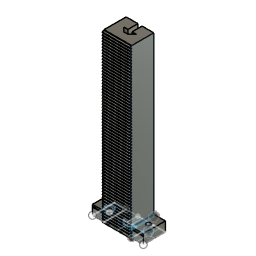
Rack_Gear_New_Version v6 (Autodesk Fusion 360 design; units mm, degrees)
description: Rack Gear; Module: 0.750000; Number of Teeth: 64; Pressure Angle: 20.000000; Root Fillet Radius: 0.032000; Clearance: 0.000000; Gear Thickness: 2.500000; Height: 2.000000;
Autodesk Fusion 360 part; units mm, degrees
(part 1 of 2)
sketch "Sketch1" plane through (0, 0, 0) normal (0, 1, 0) x (1, 0, 0) in component "Rack Gear (64 teeth)"
  line L0 (68.3534, 18.3125) -> (68.3059, 18.3125)
  arc A0 (75.3982, 18.3134) -> (75.0738, 18.5231) centre (75.3745, 18.6325) cw
  line L1 (63.641, 18.3125) -> (63.5935, 18.3125)
  arc A1 (63.5935, 18.3125) -> (63.2928, 18.5231) centre (63.5935, 18.6325) cw
  line L2 (62.7552, 20) -> (62.1231, 20)
  arc A2 (73.3665, 18.5231) -> (73.0658, 18.3125) centre (73.0658, 18.6325) cw
  arc A3 (71.0103, 18.5231) -> (70.7096, 18.3125) centre (70.7096, 18.6325) cw
  arc A4 (65.9497, 18.3125) -> (65.649, 18.5231) centre (65.9497, 18.6325) cw
  line L3 (74.5362, 20) -> (73.9041, 20)
  arc A5 (66.2979, 18.5231) -> (65.9972, 18.3125) centre (65.9972, 18.6325) cw
  line L4 (72.7176, 18.5231) -> (72.18, 20)
  arc A6 (70.6621, 18.3125) -> (70.3614, 18.5231) centre (70.6621, 18.6325) cw
  line L5 (63.2928, 18.5231) -> (62.7552, 20)
  line L6 (73.0658, 18.3125) -> (73.0183, 18.3125)
  line L7 (69.8238, 20) -> (69.1917, 20)
  line L8 (65.1114, 20) -> (64.4793, 20)
  line L9 (65.649, 18.5231) -> (65.1114, 20)
  line L10 (64.4793, 20) -> (63.9417, 18.5231)
  line L11 (70.7096, 18.3125) -> (70.6621, 18.3125)
  line L12 (68.0052, 18.5231) -> (67.4676, 20)
  arc A7 (73.0183, 18.3125) -> (72.7176, 18.5231) centre (73.0183, 18.6325) cw
  line L13 (67.4676, 20) -> (66.8355, 20)
  arc A8 (68.6541, 18.5231) -> (68.3534, 18.3125) centre (68.3534, 18.6325) cw
  line L14 (72.18, 20) -> (71.5479, 20)
  line L15 (75.0738, 18.5231) -> (74.5362, 20)
  arc A9 (68.3059, 18.3125) -> (68.0052, 18.5231) centre (68.3059, 18.6325) cw
  line L16 (71.5479, 20) -> (71.0103, 18.5231)
  line L17 (66.8355, 20) -> (66.2979, 18.5231)
  line L18 (65.9972, 18.3125) -> (65.9497, 18.3125)
  arc A10 (58.8811, 18.3125) -> (58.5804, 18.5231) centre (58.8811, 18.6325) cw
  line L19 (42.087, 18.5231) -> (41.5495, 20)
  arc A11 (63.9417, 18.5231) -> (63.641, 18.3125) centre (63.641, 18.6325) cw
  line L20 (73.9041, 20) -> (73.3665, 18.5231)
  line L21 (70.3614, 18.5231) -> (69.8238, 20)
  line L22 (69.1917, 20) -> (68.6541, 18.5231)
  line L23 (39.7308, 18.5231) -> (39.1933, 20)
  line L24 (40.9173, 20) -> (40.3798, 18.5231)
  arc A12 (49.4563, 18.3125) -> (49.1556, 18.5231) centre (49.4563, 18.6325) cw
  line L25 (58.5804, 18.5231) -> (58.0428, 20)
  arc A13 (40.0315, 18.3125) -> (39.7308, 18.5231) centre (40.0315, 18.6325) cw
  line L26 (46.2619, 20) -> (45.6297, 20)
  arc A14 (54.5169, 18.5231) -> (54.2162, 18.3125) centre (54.2162, 18.6325) cw
  line L27 (40.0791, 18.3125) -> (40.0315, 18.3125)
  line L28 (50.9743, 20) -> (50.3421, 20)
  line L29 (39.1933, 20) -> (38.5611, 20)
  arc A15 (38.0236, 18.5231) -> (37.7229, 18.3125) centre (37.7229, 18.6325) cw
  arc A16 (54.1687, 18.3125) -> (53.868, 18.5231) centre (54.1687, 18.6325) cw
  arc A17 (44.7439, 18.3125) -> (44.4432, 18.5231) centre (44.7439, 18.6325) cw
  arc A18 (37.6754, 18.3125) -> (37.3747, 18.5231) centre (37.6754, 18.6325) cw
  line L30 (37.7229, 18.3125) -> (37.6754, 18.3125)
  line L31 (55.6866, 20) -> (55.0545, 20)
  arc A19 (47.4484, 18.5231) -> (47.1477, 18.3125) centre (47.1476, 18.6325) cw
  line L32 (56.5724, 18.3125) -> (56.5249, 18.3125)
  line L33 (42.4353, 18.3125) -> (42.3877, 18.3125)
  line L34 (52.6983, 20) -> (52.1607, 18.5231)
  line L35 (53.868, 18.5231) -> (53.3304, 20)
  line L36 (57.4107, 20) -> (56.8731, 18.5231)
  line L37 (48.6181, 20) -> (47.9859, 20)
  line L38 (60.399, 20) -> (59.7669, 20)
  line L39 (43.2735, 20) -> (42.736, 18.5231)
  line L40 (45.6297, 20) -> (45.0922, 18.5231)
  arc A20 (61.2373, 18.3125) -> (60.9366, 18.5231) centre (61.2373, 18.6325) cw
  line L41 (44.4432, 18.5231) -> (43.9057, 20)
  line L42 (49.5038, 18.3125) -> (49.4563, 18.3125)
  arc A21 (42.736, 18.5231) -> (42.4353, 18.3125) centre (42.4353, 18.6325) cw
  line L43 (41.5495, 20) -> (40.9173, 20)
  line L44 (49.1556, 18.5231) -> (48.6181, 20)
  arc A22 (56.5249, 18.3125) -> (56.2242, 18.5231) centre (56.5249, 18.6325) cw
  arc A23 (51.8125, 18.3125) -> (51.5118, 18.5231) centre (51.8125, 18.6325) cw
  arc A24 (59.2293, 18.5231) -> (58.9286, 18.3125) centre (58.9286, 18.6325) cw
  line L45 (62.1231, 20) -> (61.5855, 18.5231)
  arc A25 (61.5855, 18.5231) -> (61.2848, 18.3125) centre (61.2848, 18.6325) cw
  line L46 (54.2162, 18.3125) -> (54.1687, 18.3125)
  line L47 (38.5611, 20) -> (38.0236, 18.5231)
  line L48 (51.5118, 18.5231) -> (50.9743, 20)
  line L49 (60.9366, 18.5231) -> (60.399, 20)
  line L50 (61.2848, 18.3125) -> (61.2373, 18.3125)
  line L51 (47.9859, 20) -> (47.4484, 18.5231)
  line L52 (56.2242, 18.5231) -> (55.6866, 20)
  line L53 (59.7669, 20) -> (59.2293, 18.5231)
  arc A26 (45.0922, 18.5231) -> (44.7915, 18.3125) centre (44.7915, 18.6325) cw
  arc A27 (47.1001, 18.3125) -> (46.7994, 18.5231) centre (47.1001, 18.6325) cw
  line L54 (47.1477, 18.3125) -> (47.1001, 18.3125)
  arc A28 (42.3877, 18.3125) -> (42.087, 18.5231) centre (42.3877, 18.6325) cw
  line L55 (58.9286, 18.3125) -> (58.8811, 18.3125)
  line L56 (32.1247, 20) -> (31.4926, 20)
  line L57 (51.86, 18.3125) -> (51.8125, 18.3125)
  arc A29 (40.3798, 18.5231) -> (40.0791, 18.3125) centre (40.0791, 18.6325) cw
  line L58 (44.7915, 18.3125) -> (44.7439, 18.3125)
  arc A30 (49.8045, 18.5231) -> (49.5038, 18.3125) centre (49.5038, 18.6325) cw
  line L59 (46.7994, 18.5231) -> (46.2619, 20)
  line L60 (55.0545, 20) -> (54.5169, 18.5231)
  arc A31 (52.1607, 18.5231) -> (51.86, 18.3125) centre (51.86, 18.6325) cw
  arc A32 (56.8731, 18.5231) -> (56.5724, 18.3125) centre (56.5724, 18.6325) cw
  line L61 (53.3304, 20) -> (52.6983, 20)
  line L62 (58.0428, 20) -> (57.4107, 20)
  line L63 (43.9057, 20) -> (43.2735, 20)
  line L64 (29.1364, 20) -> (28.5988, 18.5231)
  line L65 (50.3421, 20) -> (49.8045, 18.5231)
  line L66 (25.0561, 20) -> (24.424, 20)
  line L67 (24.424, 20) -> (23.8864, 18.5231)
  arc A33 (21.5302, 18.5231) -> (21.2295, 18.3125) centre (21.2295, 18.6325) cw
  arc A34 (30.955, 18.5231) -> (30.6543, 18.3125) centre (30.6543, 18.6325) cw
  line L68 (23.2375, 18.5231) -> (22.6999, 20)
  line L69 (20.8813, 18.5231) -> (20.3437, 20)
  arc A35 (35.3192, 18.3125) -> (35.0185, 18.5231) centre (35.3192, 18.6325) cw
  line L70 (37.3747, 18.5231) -> (36.8371, 20)
  line L71 (13.2751, 20) -> (12.643, 20)
  arc A36 (33.3112, 18.5231) -> (33.0105, 18.3125) centre (33.0105, 18.6325) cw
  arc A37 (14.1134, 18.3125) -> (13.8127, 18.5231) centre (14.1134, 18.6325) cw
  line L72 (28.2981, 18.3125) -> (28.2506, 18.3125)
  arc A38 (35.6674, 18.5231) -> (35.3667, 18.3125) centre (35.3667, 18.6325) cw
  line L73 (19.7116, 20) -> (19.174, 18.5231)
  arc A39 (21.182, 18.3125) -> (20.8813, 18.5231) centre (21.182, 18.6325) cw
  arc A40 (18.8258, 18.3125) -> (18.5251, 18.5231) centre (18.8258, 18.6325) cw
  line L74 (33.0105, 18.3125) -> (32.963, 18.3125)
  line L75 (26.7802, 20) -> (26.2426, 18.5231)
  arc A41 (16.8178, 18.5231) -> (16.5171, 18.3125) centre (16.5171, 18.6325) cw
  line L76 (15.6313, 20) -> (14.9992, 20)
  arc A42 (16.4696, 18.3125) -> (16.1689, 18.5231) centre (16.4696, 18.6325) cw
  arc A43 (30.6068, 18.3125) -> (30.3061, 18.5231) centre (30.6068, 18.6325) cw
  line L77 (25.9419, 18.3125) -> (25.8944, 18.3125)
  arc A44 (28.2506, 18.3125) -> (27.9499, 18.5231) centre (28.2506, 18.6325) cw
  line L78 (17.3554, 20) -> (16.8178, 18.5231)
  line L79 (36.2049, 20) -> (35.6674, 18.5231)
  line L80 (12.643, 20) -> (12.1054, 18.5231)
  line L81 (34.4809, 20) -> (33.8487, 20)
  arc A45 (25.8944, 18.3125) -> (25.5937, 18.5231) centre (25.8944, 18.6325) cw
  line L82 (35.3667, 18.3125) -> (35.3192, 18.3125)
  line L83 (29.7685, 20) -> (29.1364, 20)
  arc A46 (26.2426, 18.5231) -> (25.9419, 18.3125) centre (25.9419, 18.6325) cw
  arc A47 (12.1054, 18.5231) -> (11.8047, 18.3125) centre (11.8047, 18.6325) cw
  line L84 (23.5857, 18.3125) -> (23.5382, 18.3125)
  line L85 (33.8487, 20) -> (33.3112, 18.5231)
  line L86 (18.8733, 18.3125) -> (18.8258, 18.3125)
  line L87 (18.5251, 18.5231) -> (17.9875, 20)
  line L88 (13.8127, 18.5231) -> (13.2751, 20)
  arc A48 (23.8864, 18.5231) -> (23.5857, 18.3125) centre (23.5857, 18.6325) cw
  line L89 (16.1689, 18.5231) -> (15.6313, 20)
  line L90 (36.8371, 20) -> (36.2049, 20)
  line L91 (14.9992, 20) -> (14.4616, 18.5231)
  arc A49 (23.5382, 18.3125) -> (23.2375, 18.5231) centre (23.5382, 18.6325) cw
  line L92 (25.5937, 18.5231) -> (25.0561, 20)
  line L93 (21.2295, 18.3125) -> (21.182, 18.3125)
  line L94 (14.1609, 18.3125) -> (14.1134, 18.3125)
  line L95 (22.6999, 20) -> (22.0678, 20)
  arc A50 (32.963, 18.3125) -> (32.6623, 18.5231) centre (32.963, 18.6325) cw
  line L96 (32.6623, 18.5231) -> (32.1247, 20)
  line L97 (31.4926, 20) -> (30.955, 18.5231)
  line L98 (10.9189, 20) -> (10.2868, 20)
  arc A51 (2.6807, 18.5231) -> (2.38, 18.3125) centre (2.38, 18.6325) cw
  line L99 (30.3061, 18.5231) -> (29.7685, 20)
  line L100 (27.4123, 20) -> (26.7802, 20)
  line L101 (30.6543, 18.3125) -> (30.6068, 18.3125)
  line L102 (35.0185, 18.5231) -> (34.4809, 20)
  line L103 (22.0678, 20) -> (21.5302, 18.5231)
  arc A52 (28.5988, 18.5231) -> (28.2981, 18.3125) centre (28.2981, 18.6325) cw
  arc A53 (19.174, 18.5231) -> (18.8733, 18.3125) centre (18.8733, 18.6325) cw
  line L104 (20.3437, 20) -> (19.7116, 20)
  arc A54 (14.4616, 18.5231) -> (14.1609, 18.3125) centre (14.1609, 18.6325) cw
  line L105 (-7.9306, 20) -> (-8.5628, 20)
  arc A55 (11.7572, 18.3125) -> (11.4565, 18.5231) centre (11.7572, 18.6325) cw
  line L106 (16.5171, 18.3125) -> (16.4696, 18.3125)
  arc A56 (-9.1003, 18.5231) -> (-9.401, 18.3125) centre (-9.401, 18.6325) cw
  line L107 (-7.393, 18.5231) -> (-7.9306, 20)
  line L108 (2.38, 18.3125) -> (2.3324, 18.3125)
  line L109 (27.9499, 18.5231) -> (27.4123, 20)
  line L110 (17.9875, 20) -> (17.3554, 20)
  line L111 (10.2868, 20) -> (9.7492, 18.5231)
  line L112 (-0.862, 20) -> (-1.4942, 20)
  line L113 (-9.401, 18.3125) -> (-9.4485, 18.3125)
  arc A57 (-9.4485, 18.3125) -> (-9.7492, 18.5231) centre (-9.4485, 18.6325) cw
  arc A58 (-4.7361, 18.3125) -> (-5.0369, 18.5231) centre (-4.7361, 18.6325) cw
  line L114 (-10.2868, 20) -> (-10.9189, 20)
  arc A59 (-2.0317, 18.5231) -> (-2.3324, 18.3125) centre (-2.3324, 18.6325) cw
  line L115 (11.8047, 18.3125) -> (11.7572, 18.3125)
  line L116 (6.7441, 18.5231) -> (6.2066, 20)
  line L117 (-11.7572, 18.3125) -> (-11.8047, 18.3125)
  line L118 (7.0923, 18.3125) -> (7.0448, 18.3125)
  line L119 (-8.5628, 20) -> (-9.1003, 18.5231)
  line L120 (-7.0448, 18.3125) -> (-7.0923, 18.3125)
  line L121 (2.0317, 18.5231) -> (1.4942, 20)
  line L122 (4.7361, 18.3125) -> (4.6886, 18.3125)
  arc A60 (-0.0238, 18.3125) -> (-0.3245, 18.5231) centre (-0.0238, 18.6325) cw
  line L123 (-2.3324, 18.3125) -> (-2.38, 18.3125)
  arc A61 (9.7492, 18.5231) -> (9.4485, 18.3125) centre (9.4485, 18.6325) cw
  line L124 (-12.1054, 18.5231) -> (-12.643, 20)
  line L125 (-5.5744, 20) -> (-6.2066, 20)
  line L126 (-9.7492, 18.5231) -> (-10.2868, 20)
  line L127 (11.4565, 18.5231) -> (10.9189, 20)
  line L128 (-0.3245, 18.5231) -> (-0.862, 20)
  line L129 (-12.643, 20) -> (-13.2751, 20)
  line L130 (1.4942, 20) -> (0.862, 20)
  line L131 (-3.2182, 20) -> (-3.8504, 20)
  arc A62 (-4.3879, 18.5231) -> (-4.6886, 18.3125) centre (-4.6886, 18.6325) cw
  line L132 (-10.9189, 20) -> (-11.4565, 18.5231)
  arc A63 (-11.4565, 18.5231) -> (-11.7572, 18.3125) centre (-11.7572, 18.6325) cw
  line L133 (6.2066, 20) -> (5.5744, 20)
  arc A64 (4.6886, 18.3125) -> (4.3879, 18.5231) centre (4.6886, 18.6325) cw
  line L134 (0.0238, 18.3125) -> (-0.0238, 18.3125)
  line L135 (0.862, 20) -> (0.3245, 18.5231)
  line L136 (9.4485, 18.3125) -> (9.401, 18.3125)
  arc A65 (-11.8047, 18.3125) -> (-12.1054, 18.5231) centre (-11.8047, 18.6325) cw
  line L137 (5.5744, 20) -> (5.0369, 18.5231)
  line L138 (4.3879, 18.5231) -> (3.8504, 20)
  line L139 (3.8504, 20) -> (3.2182, 20)
  arc A66 (9.401, 18.3125) -> (9.1003, 18.5231) centre (9.401, 18.6325) cw
  line L140 (-1.4942, 20) -> (-2.0317, 18.5231)
  line L141 (7.9306, 20) -> (7.393, 18.5231)
  line L142 (-4.6886, 18.3125) -> (-4.7361, 18.3125)
  arc A67 (-6.7441, 18.5231) -> (-7.0448, 18.3125) centre (-7.0448, 18.6325) cw
  arc A68 (7.0448, 18.3125) -> (6.7441, 18.5231) centre (7.0448, 18.6325) cw
  arc A69 (7.393, 18.5231) -> (7.0923, 18.3125) centre (7.0923, 18.6325) cw
  arc A70 (0.3245, 18.5231) -> (0.0238, 18.3125) centre (0.0238, 18.6325) cw
  line L143 (-6.2066, 20) -> (-6.7441, 18.5231)
  line L144 (-3.8504, 20) -> (-4.3879, 18.5231)
  arc A71 (-7.0923, 18.3125) -> (-7.393, 18.5231) centre (-7.0923, 18.6325) cw
  arc A72 (5.0369, 18.5231) -> (4.7361, 18.3125) centre (4.7361, 18.6325) cw
  line L145 (9.1003, 18.5231) -> (8.5628, 20)
  arc A73 (-2.38, 18.3125) -> (-2.6807, 18.5231) centre (-2.38, 18.6325) cw
  line L146 (-2.6807, 18.5231) -> (-3.2182, 20)
  line L147 (-5.0369, 18.5231) -> (-5.5744, 20)
  line L148 (3.2182, 20) -> (2.6807, 18.5231)
  arc A74 (2.3324, 18.3125) -> (2.0317, 18.5231) centre (2.3324, 18.6325) cw
  line L149 (8.5628, 20) -> (7.9306, 20)
  arc A75 (-23.2375, 18.5231) -> (-23.5382, 18.3125) centre (-23.5382, 18.6325) cw
  line L150 (-19.7116, 20) -> (-20.3437, 20)
  line L151 (-25.8944, 18.3125) -> (-25.9419, 18.3125)
  arc A76 (-16.1689, 18.5231) -> (-16.4696, 18.3125) centre (-16.4696, 18.6325) cw
  line L152 (-33.3112, 18.5231) -> (-33.8487, 20)
  arc A77 (-16.5171, 18.3125) -> (-16.8178, 18.5231) centre (-16.5171, 18.6325) cw
  arc A78 (-37.7229, 18.3125) -> (-38.0236, 18.5231) centre (-37.7229, 18.6325) cw
  line L153 (-36.2049, 20) -> (-36.8371, 20)
  line L154 (-17.9875, 20) -> (-18.5251, 18.5231)
  line L155 (-26.7802, 20) -> (-27.4123, 20)
  line L156 (-20.3437, 20) -> (-20.8813, 18.5231)
  arc A79 (-27.9499, 18.5231) -> (-28.2506, 18.3125) centre (-28.2506, 18.6325) cw
  line L157 (-26.2426, 18.5231) -> (-26.7802, 20)
  arc A80 (-28.2981, 18.3125) -> (-28.5988, 18.5231) centre (-28.2981, 18.6325) cw
  line L158 (-30.6068, 18.3125) -> (-30.6543, 18.3125)
  line L159 (-21.182, 18.3125) -> (-21.2295, 18.3125)
  line L160 (-25.0561, 20) -> (-25.5937, 18.5231)
  line L161 (-34.4809, 20) -> (-35.0185, 18.5231)
  line L162 (-35.3192, 18.3125) -> (-35.3667, 18.3125)
  line L163 (-14.1134, 18.3125) -> (-14.1609, 18.3125)
  arc A81 (-20.8813, 18.5231) -> (-21.182, 18.3125) centre (-21.182, 18.6325) cw
  line L164 (-14.9992, 20) -> (-15.6313, 20)
  arc A82 (-18.8733, 18.3125) -> (-19.174, 18.5231) centre (-18.8733, 18.6325) cw
  line L165 (-23.8864, 18.5231) -> (-24.424, 20)
  arc A83 (-23.5857, 18.3125) -> (-23.8864, 18.5231) centre (-23.5857, 18.6325) cw
  arc A84 (-56.5724, 18.3125) -> (-56.8731, 18.5231) centre (-56.5724, 18.6325) cw
  arc A85 (-21.2295, 18.3125) -> (-21.5302, 18.5231) centre (-21.2295, 18.6325) cw
  line L166 (-31.4926, 20) -> (-32.1247, 20)
  line L167 (-22.6999, 20) -> (-23.2375, 18.5231)
  line L168 (-24.424, 20) -> (-25.0561, 20)
  line L169 (-15.6313, 20) -> (-16.1689, 18.5231)
  arc A86 (-25.9419, 18.3125) -> (-26.2426, 18.5231) centre (-25.9419, 18.6325) cw
  line L170 (-17.3554, 20) -> (-17.9875, 20)
  line L171 (-16.4696, 18.3125) -> (-16.5171, 18.3125)
  line L172 (-36.8371, 20) -> (-37.3747, 18.5231)
  arc A87 (-14.1609, 18.3125) -> (-14.4616, 18.5231) centre (-14.1609, 18.6325) cw
  line L173 (-13.2751, 20) -> (-13.8127, 18.5231)
  arc A88 (-30.3061, 18.5231) -> (-30.6068, 18.3125) centre (-30.6068, 18.6325) cw
  line L174 (-21.5302, 18.5231) -> (-22.0678, 20)
  line L175 (-22.0678, 20) -> (-22.6999, 20)
  line L176 (-32.963, 18.3125) -> (-33.0105, 18.3125)
  arc A89 (-13.8127, 18.5231) -> (-14.1134, 18.3125) centre (-14.1134, 18.6325) cw
  line L177 (-37.6754, 18.3125) -> (-37.7229, 18.3125)
  line L178 (-48.6181, 20) -> (-49.1556, 18.5231)
  line L179 (-59.2293, 18.5231) -> (-59.7669, 20)
  line L180 (-32.1247, 20) -> (-32.6623, 18.5231)
  line L181 (-18.8258, 18.3125) -> (-18.8733, 18.3125)
  line L182 (-45.0922, 18.5231) -> (-45.6297, 20)
  line L183 (-33.8487, 20) -> (-34.4809, 20)
  line L184 (-55.6866, 20) -> (-56.2242, 18.5231)
  arc A90 (-32.6623, 18.5231) -> (-32.963, 18.3125) centre (-32.963, 18.6325) cw
  line L185 (-23.5382, 18.3125) -> (-23.5857, 18.3125)
  line L186 (-16.8178, 18.5231) -> (-17.3554, 20)
  line L187 (-29.1364, 20) -> (-29.7685, 20)
  arc A91 (-33.0105, 18.3125) -> (-33.3112, 18.5231) centre (-33.0105, 18.6325) cw
  arc A92 (-30.6543, 18.3125) -> (-30.955, 18.5231) centre (-30.6543, 18.6325) cw
  line L188 (-14.4616, 18.5231) -> (-14.9992, 20)
  line L189 (-29.7685, 20) -> (-30.3061, 18.5231)
  line L190 (-28.5988, 18.5231) -> (-29.1364, 20)
  line L191 (-35.6674, 18.5231) -> (-36.2049, 20)
  arc A93 (-37.3747, 18.5231) -> (-37.6754, 18.3125) centre (-37.6754, 18.6325) cw
  line L192 (-28.2506, 18.3125) -> (-28.2981, 18.3125)
  arc A94 (-35.3667, 18.3125) -> (-35.6674, 18.5231) centre (-35.3667, 18.6325) cw
  line L193 (-30.955, 18.5231) -> (-31.4926, 20)
  arc A95 (-25.5937, 18.5231) -> (-25.8944, 18.3125) centre (-25.8944, 18.6325) cw
  line L194 (-19.174, 18.5231) -> (-19.7116, 20)
  arc A96 (-35.0185, 18.5231) -> (-35.3192, 18.3125) centre (-35.3192, 18.6325) cw
  line L195 (-27.4123, 20) -> (-27.9499, 18.5231)
  arc A97 (-49.5038, 18.3125) -> (-49.8045, 18.5231) centre (-49.5038, 18.6325) cw
  arc A98 (-58.9286, 18.3125) -> (-59.2293, 18.5231) centre (-58.9286, 18.6325) cw
  arc A99 (-18.5251, 18.5231) -> (-18.8258, 18.3125) centre (-18.8258, 18.6325) cw
  line L196 (-59.7669, 20) -> (-60.399, 20)
  line L197 (-54.5169, 18.5231) -> (-55.0545, 20)
  arc A100 (-60.9366, 18.5231) -> (-61.2373, 18.3125) centre (-61.2373, 18.6325) cw
  arc A101 (-58.5804, 18.5231) -> (-58.8811, 18.3125) centre (-58.8811, 18.6325) cw
  arc A102 (-42.087, 18.5231) -> (-42.3877, 18.3125) centre (-42.3877, 18.6325) cw
  arc A103 (-47.1477, 18.3125) -> (-47.4484, 18.5231) centre (-47.1476, 18.6325) cw
  line L198 (-45.6297, 20) -> (-46.2619, 20)
  arc A104 (-49.1556, 18.5231) -> (-49.4563, 18.3125) centre (-49.4563, 18.6325) cw
  arc A105 (-51.86, 18.3125) -> (-52.1607, 18.5231) centre (-51.86, 18.6325) cw
  line L199 (-54.1687, 18.3125) -> (-54.2162, 18.3125)
  line L200 (-50.9743, 20) -> (-51.5118, 18.5231)
  line L201 (-56.8731, 18.5231) -> (-57.4107, 20)
  line L202 (-58.8811, 18.3125) -> (-58.9286, 18.3125)
  arc A106 (-61.2848, 18.3125) -> (-61.5855, 18.5231) centre (-61.2848, 18.6325) cw
  line L203 (-61.2373, 18.3125) -> (-61.2848, 18.3125)
  arc A107 (-44.7915, 18.3125) -> (-45.0922, 18.5231) centre (-44.7915, 18.6325) cw
  line L204 (-52.6983, 20) -> (-53.3304, 20)
  arc A108 (-63.2928, 18.5231) -> (-63.5935, 18.3125) centre (-63.5935, 18.6325) cw
  line L205 (-43.9057, 20) -> (-44.4432, 18.5231)
  line L206 (-47.9859, 20) -> (-48.6181, 20)
  line L207 (-61.5855, 18.5231) -> (-62.1231, 20)
  line L208 (-58.0428, 20) -> (-58.5804, 18.5231)
  arc A109 (-42.4353, 18.3125) -> (-42.736, 18.5231) centre (-42.4353, 18.6325) cw
  arc A110 (-53.868, 18.5231) -> (-54.1687, 18.3125) centre (-54.1687, 18.6325) cw
  line L209 (-55.0545, 20) -> (-55.6866, 20)
  line L210 (-40.9173, 20) -> (-41.5495, 20)
  line L211 (-42.736, 18.5231) -> (-43.2735, 20)
  line L212 (-42.3877, 18.3125) -> (-42.4353, 18.3125)
  line L213 (-47.4484, 18.5231) -> (-47.9859, 20)
  line L214 (-40.0315, 18.3125) -> (-40.0791, 18.3125)
  line L215 (-41.5495, 20) -> (-42.087, 18.5231)
  line L216 (-38.0236, 18.5231) -> (-38.5611, 20)
  arc A111 (-54.2162, 18.3125) -> (-54.5169, 18.5231) centre (-54.2162, 18.6325) cw
  line L217 (-49.4563, 18.3125) -> (-49.5038, 18.3125)
  arc A112 (-56.2242, 18.5231) -> (-56.5249, 18.3125) centre (-56.5249, 18.6325) cw
  line L218 (-40.3798, 18.5231) -> (-40.9173, 20)
  line L219 (-44.7439, 18.3125) -> (-44.7915, 18.3125)
  line L220 (-52.1607, 18.5231) -> (-52.6983, 20)
  arc A113 (-39.7308, 18.5231) -> (-40.0315, 18.3125) centre (-40.0315, 18.6325) cw
  line L221 (-43.2735, 20) -> (-43.9057, 20)
  line L222 (-60.399, 20) -> (-60.9366, 18.5231)
  arc A114 (-51.5118, 18.5231) -> (-51.8125, 18.3125) centre (-51.8125, 18.6325) cw
  line L223 (-50.3421, 20) -> (-50.9743, 20)
  line L224 (-62.1231, 20) -> (-62.7552, 20)
  line L225 (-62.7552, 20) -> (-63.2928, 18.5231)
  arc A115 (-44.4432, 18.5231) -> (-44.7439, 18.3125) centre (-44.7439, 18.6325) cw
  line L226 (-49.8045, 18.5231) -> (-50.3421, 20)
  line L227 (-56.5249, 18.3125) -> (-56.5724, 18.3125)
  line L228 (-51.8125, 18.3125) -> (-51.86, 18.3125)
  line L229 (-38.5611, 20) -> (-39.1933, 20)
  arc A116 (-65.9972, 18.3125) -> (-66.2979, 18.5231) centre (-65.9972, 18.6325) cw
  line L230 (-72.18, 20) -> (-72.7176, 18.5231)
  arc A117 (-65.649, 18.5231) -> (-65.9497, 18.3125) centre (-65.9497, 18.6325) cw
  line L231 (-73.9041, 20) -> (-74.5362, 20)
  line L232 (-46.2619, 20) -> (-46.7994, 18.5231)
  line L233 (-66.2979, 18.5231) -> (-66.8355, 20)
  line L234 (-73.3665, 18.5231) -> (-73.9041, 20)
  line L235 (-73.0183, 18.3125) -> (-73.0658, 18.3125)
  arc A118 (-63.641, 18.3125) -> (-63.9417, 18.5231) centre (-63.641, 18.6325) cw
  line L236 (-70.6621, 18.3125) -> (-70.7096, 18.3125)
  line L237 (-74.5362, 20) -> (-75.0738, 18.5231)
  line L238 (-53.3304, 20) -> (-53.868, 18.5231)
  arc A119 (-75.0738, 18.5231) -> (-75.3982, 18.3134) centre (-75.3745, 18.6325) cw
  line L239 (-65.1114, 20) -> (-65.649, 18.5231)
  line L240 (-71.0103, 18.5231) -> (-71.5479, 20)
  arc A120 (-46.7994, 18.5231) -> (-47.1001, 18.3125) centre (-47.1001, 18.6325) cw
  arc A121 (-70.7096, 18.3125) -> (-71.0103, 18.5231) centre (-70.7096, 18.6325) cw
  line L241 (-47.1001, 18.3125) -> (-47.1477, 18.3125)
  line L242 (-63.5935, 18.3125) -> (-63.641, 18.3125)
  line L243 (-67.4676, 20) -> (-68.0052, 18.5231)
  line L244 (-68.6541, 18.5231) -> (-69.1917, 20)
  line L245 (-69.8238, 20) -> (-70.3614, 18.5231)
  line L246 (-63.9417, 18.5231) -> (-64.4793, 20)
  line L247 (-64.4793, 20) -> (-65.1114, 20)
  line L248 (-75.3982, 0) -> (75.3982, 0)
  line L249 (-65.9497, 18.3125) -> (-65.9972, 18.3125)
  arc A122 (-68.3534, 18.3125) -> (-68.6541, 18.5231) centre (-68.3534, 18.6325) cw
  arc A123 (-68.0052, 18.5231) -> (-68.3059, 18.3125) centre (-68.3059, 18.6325) cw
  line L250 (-69.1917, 20) -> (-69.8238, 20)
  line L251 (-57.4107, 20) -> (-58.0428, 20)
  line L252 (-71.5479, 20) -> (-72.18, 20)
  line L253 (-39.1933, 20) -> (-39.7308, 18.5231)
  arc A124 (-73.0658, 18.3125) -> (-73.3665, 18.5231) centre (-73.0658, 18.6325) cw
  arc A125 (-40.0791, 18.3125) -> (-40.3798, 18.5231) centre (-40.0791, 18.6325) cw
  line L254 (-66.8355, 20) -> (-67.4676, 20)
  arc A126 (-72.7176, 18.5231) -> (-73.0183, 18.3125) centre (-73.0183, 18.6325) cw
  line L255 (-75.3982, 18.3134) -> (-75.3982, 0)
  line L256 (-68.3059, 18.3125) -> (-68.3534, 18.3125)
  arc A127 (-70.3614, 18.5231) -> (-70.6621, 18.3125) centre (-70.6621, 18.6325) cw
  line L257 (75.3982, 0) -> (75.3982, 18.3134)
extrude "Extrude1" add sketch "Sketch1" along normal blind 25 makes body 1 in component "Rack Gear (64 teeth)"
sketch "Sketch2" plane through (0, 0, 0) normal (0, 1, 0) x (1, 0, 0) in component "Rack Gear (64 teeth)"
  line L0 (-75.4082, 19.25) -> (75.4082, 19.25) construction
extrude "Extrude2" add 1 faces at (-25.1327, 16.6667, 0) along direction (0, 0, 1) blind 1.687 on bodies 1 bodies 1 in component "Rack Gear (64 teeth)"
sketch "Sketch1 (2)" plane through (0, 0, -86.9185) normal (0, 0, -1) x (1, 0, 0)
  line L0 (12.5, -25.7073) -> (12.5, -5.707)
  line L1 (12.5, -5.707) -> (-12.5, -5.707)
  line L2 (-12.5, -5.707) -> (-12.5, -25.7073)
  line L3 (-12.5, -25.7073) -> (12.5, -25.7073)
  line L4 (12.5, -5.707) -> (-12.5, -5.707) construction
  line L5 (-12.5, -5.707) -> (-12.5, -25.7073) construction
  line L6 (-12.5, -25.7073) -> (12.5, -25.7073) construction
  line L7 (12.5, -25.7073) -> (12.5, -5.707) construction
  line L8 (0, -25.7073) -> (0, -5.707)
  line L9 (-12.5, -15.7072) -> (12.5, -15.7072)
  line L10 (23, -25.7073) -> (23, -5.707) construction
  line L11 (12.5, -5.707) -> (23, -5.707)
  line L12 (23, -5.707) -> (23, -25.7073)
  line L13 (23, -25.7073) -> (12.5, -25.7073)
  line L14 (12.5, -25.7073) -> (12.5, -5.707)
  line L15 (-12.5, -5.707) -> (-23, -5.707)
  line L16 (-23, -25.7073) -> (-23, -5.707) construction
  line L17 (-23, -25.7073) -> (-12.5, -25.7073)
  line L18 (-12.5, -25.7073) -> (-12.5, -5.707)
  line L19 (17.75, -5.707) -> (17.75, -25.7073)
  line L20 (12.5, -15.7072) -> (23, -15.7072)
  circle A0 centre (17.75, -15.7072) radius 2
  circle A1 centre (-17.75, -15.7072) radius 2
  line L21 (-23, -25.7073) -> (-23, -5.707)
  line L22 (0, -25.7073) -> (1.875, -25.7073) construction
  line L23 (1.875, -25.7073) -> (1.875, -16.7073)
  line L24 (-1.875, -25.7073) -> (-1.875, -16.7073)
  line L25 (1.875, -16.7073) -> (5.625, -16.7073)
  line L26 (-1.875, -16.7073) -> (-5.625, -16.7073)
  line L27 (1.875, -12.9573) -> (-1.875, -12.9573)
  line L28 (5.625, -16.7073) -> (1.875, -12.9573)
  line L29 (-5.625, -16.7073) -> (-1.875, -12.9573)
  dimension "d7" = 10.5
  dimension "d8" = 4
  dimension "d24" = 1.875
  dimension "d25" = 9
  dimension "d26" = 3.75
  dimension "d27" = 3.75
  dimension "d29" = 3.75
  constraint horizontal L4
  constraint vertical L5
  constraint horizontal L6
  constraint vertical L7
  constraint coincident L2.end L3.start
  constraint coincident L0.end L1.start
  constraint midpoint L6 L8.start
  constraint midpoint L4 L8.end
  constraint midpoint L5 L9.start
  constraint midpoint L7 L9.end
  constraint horizontal L11
  constraint vertical L12
  constraint horizontal L13
  constraint vertical L14
  constraint symmetric L0.end L8 L1.end
  constraint symmetric L8 L10.start L16.start
  constraint symmetric L8 L10.end L15.end
  constraint symmetric L8 L0.start L2.end
  constraint midpoint L11 L19.start
  constraint midpoint L13 L19.end
  constraint midpoint L10 L20.end
  constraint perpendicular L10 L20
  constraint midpoint L20 A0.centre
  constraint symmetric L8 A0 A1
  constraint perpendicular L8 L22
  constraint perpendicular L6 L23
  constraint symmetric L8 L22.end L24.start
  constraint symmetric L8 L23.end L24.end
  constraint perpendicular L23 L25
  constraint perpendicular L24 L26
  constraint perpendicular L28 L29
  measures "d8" diameter of A0
  measures "d24" distance of L8.start L22.end
  measures "d25" distance of L22.end L23.end
  measures "d26" distance of L23.end L25.end
  measures "d27" distance of L24.end L26.end
  measures "d29" distance of L27.start L27.end
extrude "Extrude1'" add sketch "Sketch1 (2)" against normal blind 3.1 separate body contours L0 L13 L14 L19 L20 A0 | L0 L11 L14 L19 L20 A0 | L12 L13 L19 L20 A0 | L11 L12 L19 L20 A0 | L2 L15 L17 L18 L21 makes body 2 at (17.7002, 23.0388, -83.8185) makes body 3 at (-17.7002, 8.3756, -86.9185)
sketch "Sketch2 (2)" plane through (0, 0, -83.8185) normal (0, 0, 1) x (-1, 0, 0)
  circle A0 centre (-17.75, -15.7072) radius 2
  line L0 (-23, -25.7073) -> (-12.5, -25.7073)
  line L1 (-12.5, -25.7073) -> (-12.5, -5.707)
  line L2 (-12.5, -5.707) -> (-23, -5.707)
  line L3 (-23, -5.707) -> (-23, -25.7073)
  line L4 (-19.6264, -12.4572) -> (-21.5028, -15.7072)
  line L5 (-21.5028, -15.7072) -> (-19.6264, -18.9572)
  line L6 (-19.6264, -18.9572) -> (-15.8736, -18.9572)
  line L7 (-15.8736, -18.9572) -> (-13.9972, -15.7072)
  line L8 (-13.9972, -15.7072) -> (-15.8736, -12.4572)
  line L9 (-15.8736, -12.4572) -> (-19.6264, -12.4572)
  point P0 (-17.75, -15.7072)
  dimension "d11" = 3.25
  constraint coincident P0 A0.centre
  measures "d11" distance of P0 L9
sketch "Sketch3" plane through (0, 0, -83.8185) normal (0, 0, 1) x (-1, 0, 0)
  circle A0 centre (17.75, -15.7072) radius 2
  line L0 (12.5, -5.707) -> (12.5, -25.7073)
  line L1 (12.5, -25.7073) -> (23, -25.7073)
  line L2 (23, -25.7073) -> (23, -5.707)
  line L3 (23, -5.707) -> (12.5, -5.707)
  line L4 (15.8736, -12.4572) -> (13.9972, -15.7072)
  line L5 (13.9972, -15.7072) -> (15.8736, -18.9572)
  line L6 (15.8736, -18.9572) -> (19.6264, -18.9572)
  line L7 (19.6264, -18.9572) -> (21.5028, -15.7072)
  line L8 (21.5028, -15.7072) -> (19.6264, -12.4572)
  line L9 (19.6264, -12.4572) -> (15.8736, -12.4572)
  point P0 (17.75, -15.7072)
  dimension "d12" = 3.25
  constraint coincident P0 A0.centre
  measures "d12" distance of P0 L9
extrude "Extrude2'" add sketch "Sketch2 (2)" sketch "Sketch3" along normal blind 3.4 contours L0 L1 L2 L3 of sketch 2 contours L0 L1 L2 L3 bodies 2 3
sketch "Sketch4" plane through (12.5, 0, 0) normal (1, 0, 0) x (0, 1, 0)
  line L0 (5.707, -86.9185) -> (25.7073, -86.9185)
  line L1 (25.7073, -86.9185) -> (25.7073, 63.8778)
  line L2 (25.7073, 63.8778) -> (5.707, 63.8778)
  arc A0 (5.4973, 63.5534) -> (5.707, 63.8778) centre (5.3878, 63.8541) ccw
  line L3 (5.4973, 63.5534) -> (4.0203, 63.0158)
  line L4 (4.0203, 63.0158) -> (4.0203, 62.3837)
  line L5 (4.0203, 62.3837) -> (5.4973, 61.8461)
  arc A1 (5.7078, 61.5454) -> (5.4973, 61.8461) centre (5.3878, 61.5454) ccw
  line L6 (5.7078, 61.5454) -> (5.7078, 61.4979)
  arc A2 (5.4973, 61.1972) -> (5.7078, 61.4979) centre (5.3878, 61.4979) ccw
  line L7 (5.4973, 61.1972) -> (4.0203, 60.6597)
  line L8 (4.0203, 60.6597) -> (4.0203, 60.0275)
  line L9 (4.0203, 60.0275) -> (5.4973, 59.4899)
  arc A3 (5.7078, 59.1892) -> (5.4973, 59.4899) centre (5.3878, 59.1892) ccw
  line L10 (5.7078, 59.1892) -> (5.7078, 59.1417)
  arc A4 (5.4973, 58.841) -> (5.7078, 59.1417) centre (5.3878, 59.1417) ccw
  line L11 (5.4973, 58.841) -> (4.0203, 58.3035)
  line L12 (4.0203, 58.3035) -> (4.0203, 57.6713)
  line L13 (4.0203, 57.6713) -> (5.4973, 57.1338)
  arc A5 (5.7078, 56.8331) -> (5.4973, 57.1338) centre (5.3878, 56.8331) ccw
  line L14 (5.7078, 56.8331) -> (5.7078, 56.7855)
  arc A6 (5.4973, 56.4848) -> (5.7078, 56.7855) centre (5.3878, 56.7855) ccw
  line L15 (5.4973, 56.4848) -> (4.0203, 55.9473)
  line L16 (4.0203, 55.9473) -> (4.0203, 55.3151)
  line L17 (4.0203, 55.3151) -> (5.4973, 54.7776)
  arc A7 (5.7078, 54.4769) -> (5.4973, 54.7776) centre (5.3878, 54.4769) ccw
  line L18 (5.7078, 54.4769) -> (5.7078, 54.4293)
  arc A8 (5.4973, 54.1286) -> (5.7078, 54.4293) centre (5.3878, 54.4293) ccw
  line L19 (5.4973, 54.1286) -> (4.0203, 53.5911)
  line L20 (4.0203, 53.5911) -> (4.0203, 52.9589)
  line L21 (4.0203, 52.9589) -> (5.4973, 52.4214)
  arc A9 (5.7078, 52.1207) -> (5.4973, 52.4214) centre (5.3878, 52.1207) ccw
  line L22 (5.7078, 52.1207) -> (5.7078, 52.0731)
  arc A10 (5.4973, 51.7724) -> (5.7078, 52.0731) centre (5.3878, 52.0731) ccw
  line L23 (5.4973, 51.7724) -> (4.0203, 51.2349)
  line L24 (4.0203, 51.2349) -> (4.0203, 50.6027)
  line L25 (4.0203, 50.6027) -> (5.4973, 50.0652)
  arc A11 (5.7078, 49.7645) -> (5.4973, 50.0652) centre (5.3878, 49.7645) ccw
  line L26 (5.7078, 49.7645) -> (5.7078, 49.7169)
  arc A12 (5.4973, 49.4162) -> (5.7078, 49.7169) centre (5.3878, 49.7169) ccw
  line L27 (5.4973, 49.4162) -> (4.0203, 48.8787)
  line L28 (4.0203, 48.8787) -> (4.0203, 48.2465)
  line L29 (4.0203, 48.2465) -> (5.4973, 47.709)
  arc A13 (5.7078, 47.4083) -> (5.4973, 47.709) centre (5.3878, 47.4083) ccw
  line L30 (5.7078, 47.4083) -> (5.7078, 47.3608)
  arc A14 (5.4973, 47.0601) -> (5.7078, 47.3608) centre (5.3878, 47.3608) ccw
  line L31 (5.4973, 47.0601) -> (4.0203, 46.5225)
  line L32 (4.0203, 46.5225) -> (4.0203, 45.8903)
  line L33 (4.0203, 45.8903) -> (5.4973, 45.3528)
  arc A15 (5.7078, 45.0521) -> (5.4973, 45.3528) centre (5.3878, 45.0521) ccw
  line L34 (5.7078, 45.0521) -> (5.7078, 45.0046)
  arc A16 (5.4973, 44.7039) -> (5.7078, 45.0046) centre (5.3878, 45.0046) ccw
  line L35 (5.4973, 44.7039) -> (4.0203, 44.1663)
  line L36 (4.0203, 44.1663) -> (4.0203, 43.5342)
  line L37 (4.0203, 43.5342) -> (5.4973, 42.9966)
  arc A17 (5.7078, 42.6959) -> (5.4973, 42.9966) centre (5.3878, 42.6959) ccw
  line L38 (5.7078, 42.6959) -> (5.7078, 42.6484)
  arc A18 (5.4973, 42.3477) -> (5.7078, 42.6484) centre (5.3878, 42.6484) ccw
  line L39 (5.4973, 42.3477) -> (4.0203, 41.8101)
  line L40 (4.0203, 41.8101) -> (4.0203, 41.178)
  line L41 (4.0203, 41.178) -> (5.4973, 40.6404)
  arc A19 (5.7078, 40.3397) -> (5.4973, 40.6404) centre (5.3878, 40.3397) ccw
  line L42 (5.7078, 40.3397) -> (5.7078, 40.2922)
  arc A20 (5.4973, 39.9915) -> (5.7078, 40.2922) centre (5.3878, 40.2922) ccw
  line L43 (5.4973, 39.9915) -> (4.0203, 39.4539)
  line L44 (4.0203, 39.4539) -> (4.0203, 38.8218)
  line L45 (4.0203, 38.8218) -> (5.4973, 38.2842)
  arc A21 (5.7078, 37.9835) -> (5.4973, 38.2842) centre (5.3878, 37.9835) ccw
  line L46 (5.7078, 37.9835) -> (5.7078, 37.936)
  arc A22 (5.4973, 37.6353) -> (5.7078, 37.936) centre (5.3878, 37.936) ccw
  line L47 (5.4973, 37.6353) -> (4.0203, 37.0977)
  line L48 (4.0203, 37.0977) -> (4.0203, 36.4656)
  line L49 (4.0203, 36.4656) -> (5.4973, 35.928)
  arc A23 (5.7078, 35.6273) -> (5.4973, 35.928) centre (5.3878, 35.6273) ccw
  line L50 (5.7078, 35.6273) -> (5.7078, 35.5798)
  arc A24 (5.4973, 35.2791) -> (5.7078, 35.5798) centre (5.3878, 35.5798) ccw
  line L51 (5.4973, 35.2791) -> (4.0203, 34.7415)
  line L52 (4.0203, 34.7415) -> (4.0203, 34.1094)
  line L53 (4.0203, 34.1094) -> (5.4973, 33.5718)
  arc A25 (5.7078, 33.2711) -> (5.4973, 33.5718) centre (5.3878, 33.2711) ccw
  line L54 (5.7078, 33.2711) -> (5.7078, 33.2236)
  arc A26 (5.4973, 32.9229) -> (5.7078, 33.2236) centre (5.3878, 33.2236) ccw
  line L55 (5.4973, 32.9229) -> (4.0203, 32.3853)
  line L56 (4.0203, 32.3853) -> (4.0203, 31.7532)
  line L57 (4.0203, 31.7532) -> (5.4973, 31.2156)
  arc A27 (5.7078, 30.9149) -> (5.4973, 31.2156) centre (5.3878, 30.9149) ccw
  line L58 (5.7078, 30.9149) -> (5.7078, 30.8674)
  arc A28 (5.4973, 30.5667) -> (5.7078, 30.8674) centre (5.3878, 30.8674) ccw
  line L59 (5.4973, 30.5667) -> (4.0203, 30.0291)
  line L60 (4.0203, 30.0291) -> (4.0203, 29.397)
  line L61 (4.0203, 29.397) -> (5.4973, 28.8594)
  arc A29 (5.7078, 28.5587) -> (5.4973, 28.8594) centre (5.3878, 28.5587) ccw
  line L62 (5.7078, 28.5587) -> (5.7078, 28.5112)
  arc A30 (5.4973, 28.2105) -> (5.7078, 28.5112) centre (5.3878, 28.5112) ccw
  line L63 (5.4973, 28.2105) -> (4.0203, 27.6729)
  line L64 (4.0203, 27.6729) -> (4.0203, 27.0408)
  line L65 (4.0203, 27.0408) -> (5.4973, 26.5032)
  arc A31 (5.7078, 26.2025) -> (5.4973, 26.5032) centre (5.3878, 26.2025) ccw
  line L66 (5.7078, 26.2025) -> (5.7078, 26.155)
  arc A32 (5.4973, 25.8543) -> (5.7078, 26.155) centre (5.3878, 26.155) ccw
  line L67 (5.4973, 25.8543) -> (4.0203, 25.3167)
  line L68 (4.0203, 25.3167) -> (4.0203, 24.6846)
  line L69 (4.0203, 24.6846) -> (5.4973, 24.147)
  arc A33 (5.7078, 23.8463) -> (5.4973, 24.147) centre (5.3878, 23.8463) ccw
  line L70 (5.7078, 23.8463) -> (5.7078, 23.7988)
  arc A34 (5.4973, 23.4981) -> (5.7078, 23.7988) centre (5.3878, 23.7988) ccw
  line L71 (5.4973, 23.4981) -> (4.0203, 22.9605)
  line L72 (4.0203, 22.9605) -> (4.0203, 22.3284)
  line L73 (4.0203, 22.3284) -> (5.4973, 21.7908)
  arc A35 (5.7078, 21.4901) -> (5.4973, 21.7908) centre (5.3878, 21.4901) ccw
  line L74 (5.7078, 21.4901) -> (5.7078, 21.4426)
  arc A36 (5.4973, 21.1419) -> (5.7078, 21.4426) centre (5.3878, 21.4426) ccw
  line L75 (5.4973, 21.1419) -> (4.0203, 20.6043)
  line L76 (4.0203, 20.6043) -> (4.0203, 19.9722)
  line L77 (4.0203, 19.9722) -> (5.4973, 19.4346)
  arc A37 (5.7078, 19.1339) -> (5.4973, 19.4346) centre (5.3878, 19.1339) ccw
  line L78 (5.7078, 19.1339) -> (5.7078, 19.0864)
  arc A38 (5.4973, 18.7857) -> (5.7078, 19.0864) centre (5.3878, 19.0864) ccw
  line L79 (5.4973, 18.7857) -> (4.0203, 18.2482)
  line L80 (4.0203, 18.2482) -> (4.0203, 17.616)
  line L81 (4.0203, 17.616) -> (5.4973, 17.0784)
  arc A39 (5.7078, 16.7777) -> (5.4973, 17.0784) centre (5.3878, 16.7777) ccw
  line L82 (5.7078, 16.7777) -> (5.7078, 16.7302)
  arc A40 (5.4973, 16.4295) -> (5.7078, 16.7302) centre (5.3878, 16.7302) ccw
  line L83 (5.4973, 16.4295) -> (4.0203, 15.892)
  line L84 (4.0203, 15.892) -> (4.0203, 15.2598)
  line L85 (4.0203, 15.2598) -> (5.4973, 14.7223)
  arc A41 (5.7078, 14.4216) -> (5.4973, 14.7223) centre (5.3878, 14.4216) ccw
  line L86 (5.7078, 14.4216) -> (5.7078, 14.374)
  arc A42 (5.4973, 14.0733) -> (5.7078, 14.374) centre (5.3878, 14.374) ccw
  line L87 (5.4973, 14.0733) -> (4.0203, 13.5358)
  line L88 (4.0203, 13.5358) -> (4.0203, 12.9036)
  line L89 (4.0203, 12.9036) -> (5.4973, 12.3661)
  arc A43 (5.7078, 12.0654) -> (5.4973, 12.3661) centre (5.3878, 12.0654) ccw
  line L90 (5.7078, 12.0654) -> (5.7078, 12.0178)
  arc A44 (5.4973, 11.7171) -> (5.7078, 12.0178) centre (5.3878, 12.0178) ccw
  line L91 (5.4973, 11.7171) -> (4.0203, 11.1796)
  line L92 (4.0203, 11.1796) -> (4.0203, 10.5474)
  line L93 (4.0203, 10.5474) -> (5.4973, 10.0099)
  arc A45 (5.7078, 9.7092) -> (5.4973, 10.0099) centre (5.3878, 9.7092) ccw
  line L94 (5.7078, 9.7092) -> (5.7078, 9.6616)
  arc A46 (5.4973, 9.3609) -> (5.7078, 9.6616) centre (5.3878, 9.6616) ccw
  line L95 (5.4973, 9.3609) -> (4.0203, 8.8234)
  line L96 (4.0203, 8.8234) -> (4.0203, 8.1912)
  line L97 (4.0203, 8.1912) -> (5.4973, 7.6537)
  arc A47 (5.7078, 7.353) -> (5.4973, 7.6537) centre (5.3878, 7.353) ccw
  line L98 (5.7078, 7.353) -> (5.7078, 7.3054)
  arc A48 (5.4973, 7.0047) -> (5.7078, 7.3054) centre (5.3878, 7.3054) ccw
  line L99 (5.4973, 7.0047) -> (4.0203, 6.4672)
  line L100 (4.0203, 6.4672) -> (4.0203, 5.835)
  line L101 (4.0203, 5.835) -> (5.4973, 5.2975)
  arc A49 (5.7078, 4.9968) -> (5.4973, 5.2975) centre (5.3878, 4.9968) ccw
  line L102 (5.7078, 4.9968) -> (5.7078, 4.9493)
  arc A50 (5.4973, 4.6486) -> (5.7078, 4.9493) centre (5.3878, 4.9493) ccw
  line L103 (5.4973, 4.6486) -> (4.0203, 4.111)
  line L104 (4.0203, 4.111) -> (4.0203, 3.4788)
  line L105 (4.0203, 3.4788) -> (5.4973, 2.9413)
  arc A51 (5.7078, 2.6406) -> (5.4973, 2.9413) centre (5.3878, 2.6406) ccw
  line L106 (5.7078, 2.6406) -> (5.7078, 2.5931)
  arc A52 (5.4973, 2.2924) -> (5.7078, 2.5931) centre (5.3878, 2.5931) ccw
  line L107 (5.4973, 2.2924) -> (4.0203, 1.7548)
  line L108 (4.0203, 1.7548) -> (4.0203, 1.1226)
  line L109 (4.0203, 1.1226) -> (5.4973, 0.5851)
  arc A53 (5.7078, 0.2844) -> (5.4973, 0.5851) centre (5.3878, 0.2844) ccw
  line L110 (5.7078, 0.2844) -> (5.7078, 0.2369)
  arc A54 (5.4973, -0.0638) -> (5.7078, 0.2369) centre (5.3878, 0.2369) ccw
  line L111 (5.4973, -0.0638) -> (4.0203, -0.6014)
  line L112 (4.0203, -0.6014) -> (4.0203, -1.2335)
  line L113 (4.0203, -1.2335) -> (5.4973, -1.7711)
  arc A55 (5.7078, -2.0718) -> (5.4973, -1.7711) centre (5.3878, -2.0718) ccw
  line L114 (5.7078, -2.0718) -> (5.7078, -2.1193)
  arc A56 (5.4973, -2.42) -> (5.7078, -2.1193) centre (5.3878, -2.1193) ccw
  line L115 (5.4973, -2.42) -> (4.0203, -2.9576)
  line L116 (4.0203, -2.9576) -> (4.0203, -3.5897)
  line L117 (4.0203, -3.5897) -> (5.4973, -4.1273)
  arc A57 (5.7078, -4.428) -> (5.4973, -4.1273) centre (5.3878, -4.428) ccw
  line L118 (5.7078, -4.428) -> (5.7078, -4.4755)
  arc A58 (5.4973, -4.7762) -> (5.7078, -4.4755) centre (5.3878, -4.4755) ccw
  line L119 (5.4973, -4.7762) -> (4.0203, -5.3138)
  line L120 (4.0203, -5.3138) -> (4.0203, -5.9459)
  line L121 (4.0203, -5.9459) -> (5.4973, -6.4835)
  arc A59 (5.7078, -6.7842) -> (5.4973, -6.4835) centre (5.3878, -6.7842) ccw
  line L122 (5.7078, -6.7842) -> (5.7078, -6.8317)
  arc A60 (5.4973, -7.1324) -> (5.7078, -6.8317) centre (5.3878, -6.8317) ccw
  line L123 (5.4973, -7.1324) -> (4.0203, -7.67)
  line L124 (4.0203, -7.67) -> (4.0203, -8.3021)
  line L125 (4.0203, -8.3021) -> (5.4973, -8.8397)
  arc A61 (5.7078, -9.1404) -> (5.4973, -8.8397) centre (5.3878, -9.1404) ccw
  line L126 (5.7078, -9.1404) -> (5.7078, -9.1879)
  arc A62 (5.4973, -9.4886) -> (5.7078, -9.1879) centre (5.3878, -9.1879) ccw
  line L127 (5.4973, -9.4886) -> (4.0203, -10.0262)
  line L128 (4.0203, -10.0262) -> (4.0203, -10.6583)
  line L129 (4.0203, -10.6583) -> (5.4973, -11.1959)
  arc A63 (5.7078, -11.4966) -> (5.4973, -11.1959) centre (5.3878, -11.4966) ccw
  line L130 (5.7078, -11.4966) -> (5.7078, -11.5441)
  arc A64 (5.4973, -11.8448) -> (5.7078, -11.5441) centre (5.3878, -11.5441) ccw
  line L131 (5.4973, -11.8448) -> (4.0203, -12.3824)
  line L132 (4.0203, -12.3824) -> (4.0203, -13.0145)
  line L133 (4.0203, -13.0145) -> (5.4973, -13.5521)
  arc A65 (5.7078, -13.8528) -> (5.4973, -13.5521) centre (5.3878, -13.8528) ccw
  line L134 (5.7078, -13.8528) -> (5.7078, -13.9003)
  arc A66 (5.4973, -14.201) -> (5.7078, -13.9003) centre (5.3878, -13.9003) ccw
  line L135 (5.4973, -14.201) -> (4.0203, -14.7386)
  line L136 (4.0203, -14.7386) -> (4.0203, -15.3707)
  line L137 (4.0203, -15.3707) -> (5.4973, -15.9083)
  arc A67 (5.7078, -16.209) -> (5.4973, -15.9083) centre (5.3878, -16.209) ccw
  line L138 (5.7078, -16.209) -> (5.7078, -16.2565)
  arc A68 (5.4973, -16.5572) -> (5.7078, -16.2565) centre (5.3878, -16.2565) ccw
  line L139 (5.4973, -16.5572) -> (4.0203, -17.0948)
  line L140 (4.0203, -17.0948) -> (4.0203, -17.7269)
  line L141 (4.0203, -17.7269) -> (5.4973, -18.2645)
  arc A69 (5.7078, -18.5652) -> (5.4973, -18.2645) centre (5.3878, -18.5652) ccw
  line L142 (5.7078, -18.5652) -> (5.7078, -18.6127)
  arc A70 (5.4973, -18.9134) -> (5.7078, -18.6127) centre (5.3878, -18.6127) ccw
  line L143 (5.4973, -18.9134) -> (4.0203, -19.451)
  line L144 (4.0203, -19.451) -> (4.0203, -20.0831)
  line L145 (4.0203, -20.0831) -> (5.4973, -20.6207)
  arc A71 (5.7078, -20.9214) -> (5.4973, -20.6207) centre (5.3878, -20.9214) ccw
  line L146 (5.7078, -20.9214) -> (5.7078, -20.9689)
  arc A72 (5.4973, -21.2696) -> (5.7078, -20.9689) centre (5.3878, -20.9689) ccw
  line L147 (5.4973, -21.2696) -> (4.0203, -21.8072)
  line L148 (4.0203, -21.8072) -> (4.0203, -22.4393)
  line L149 (4.0203, -22.4393) -> (5.4973, -22.9769)
  arc A73 (5.7078, -23.2776) -> (5.4973, -22.9769) centre (5.3878, -23.2776) ccw
  line L150 (5.7078, -23.2776) -> (5.7078, -23.3251)
  arc A74 (5.4973, -23.6258) -> (5.7078, -23.3251) centre (5.3878, -23.3251) ccw
  line L151 (5.4973, -23.6258) -> (4.0203, -24.1633)
  line L152 (4.0203, -24.1633) -> (4.0203, -24.7955)
  line L153 (4.0203, -24.7955) -> (5.4973, -25.3331)
  arc A75 (5.7078, -25.6338) -> (5.4973, -25.3331) centre (5.3878, -25.6338) ccw
  line L154 (5.7078, -25.6338) -> (5.7078, -25.6813)
  arc A76 (5.4973, -25.982) -> (5.7078, -25.6813) centre (5.3878, -25.6813) ccw
  line L155 (5.4973, -25.982) -> (4.0203, -26.5195)
  line L156 (4.0203, -26.5195) -> (4.0203, -27.1517)
  line L157 (4.0203, -27.1517) -> (5.4973, -27.6892)
  arc A77 (5.7078, -27.9899) -> (5.4973, -27.6892) centre (5.3878, -27.99) ccw
  line L158 (5.7078, -27.9899) -> (5.7078, -28.0375)
  arc A78 (5.4973, -28.3382) -> (5.7078, -28.0375) centre (5.3878, -28.0375) ccw
  line L159 (5.4973, -28.3382) -> (4.0203, -28.8757)
  line L160 (4.0203, -28.8757) -> (4.0203, -29.5079)
  line L161 (4.0203, -29.5079) -> (5.4973, -30.0454)
  arc A79 (5.7078, -30.3461) -> (5.4973, -30.0454) centre (5.3878, -30.3461) ccw
  line L162 (5.7078, -30.3461) -> (5.7078, -30.3937)
  arc A80 (5.4973, -30.6944) -> (5.7078, -30.3937) centre (5.3878, -30.3937) ccw
  line L163 (5.4973, -30.6944) -> (4.0203, -31.2319)
  line L164 (4.0203, -31.2319) -> (4.0203, -31.8641)
  line L165 (4.0203, -31.8641) -> (5.4973, -32.4016)
  arc A81 (5.7078, -32.7023) -> (5.4973, -32.4016) centre (5.3878, -32.7023) ccw
  line L166 (5.7078, -32.7023) -> (5.7078, -32.7499)
  arc A82 (5.4973, -33.0506) -> (5.7078, -32.7499) centre (5.3878, -32.7499) ccw
  line L167 (5.4973, -33.0506) -> (4.0203, -33.5881)
  line L168 (4.0203, -33.5881) -> (4.0203, -34.2203)
  line L169 (4.0203, -34.2203) -> (5.4973, -34.7578)
  arc A83 (5.7078, -35.0585) -> (5.4973, -34.7578) centre (5.3878, -35.0585) ccw
  line L170 (5.7078, -35.0585) -> (5.7078, -35.1061)
  arc A84 (5.4973, -35.4068) -> (5.7078, -35.1061) centre (5.3878, -35.1061) ccw
  line L171 (5.4973, -35.4068) -> (4.0203, -35.9443)
  line L172 (4.0203, -35.9443) -> (4.0203, -36.5765)
  line L173 (4.0203, -36.5765) -> (5.4973, -37.114)
  arc A85 (5.7078, -37.4147) -> (5.4973, -37.114) centre (5.3878, -37.4147) ccw
  line L174 (5.7078, -37.4147) -> (5.7078, -37.4622)
  arc A86 (5.4973, -37.7629) -> (5.7078, -37.4622) centre (5.3878, -37.4622) ccw
  line L175 (5.4973, -37.7629) -> (4.0203, -38.3005)
  line L176 (4.0203, -38.3005) -> (4.0203, -38.9327)
  line L177 (4.0203, -38.9327) -> (5.4973, -39.4702)
  arc A87 (5.7078, -39.7709) -> (5.4973, -39.4702) centre (5.3878, -39.7709) ccw
  line L178 (5.7078, -39.7709) -> (5.7078, -39.8184)
  arc A88 (5.4973, -40.1191) -> (5.7078, -39.8184) centre (5.3878, -39.8184) ccw
  line L179 (5.4973, -40.1191) -> (4.0203, -40.6567)
  line L180 (4.0203, -40.6567) -> (4.0203, -41.2889)
  line L181 (4.0203, -41.2889) -> (5.4973, -41.8264)
  arc A89 (5.7078, -42.1271) -> (5.4973, -41.8264) centre (5.3878, -42.1271) ccw
  line L182 (5.7078, -42.1271) -> (5.7078, -42.1746)
  arc A90 (5.4973, -42.4753) -> (5.7078, -42.1746) centre (5.3878, -42.1746) ccw
  line L183 (5.4973, -42.4753) -> (4.0203, -43.0129)
  line L184 (4.0203, -43.0129) -> (4.0203, -43.645)
  line L185 (4.0203, -43.645) -> (5.4973, -44.1826)
  arc A91 (5.7078, -44.4833) -> (5.4973, -44.1826) centre (5.3878, -44.4833) ccw
  line L186 (5.7078, -44.4833) -> (5.7078, -44.5308)
  arc A92 (5.4973, -44.8315) -> (5.7078, -44.5308) centre (5.3878, -44.5308) ccw
  line L187 (5.4973, -44.8315) -> (4.0203, -45.3691)
  line L188 (4.0203, -45.3691) -> (4.0203, -46.0012)
  line L189 (4.0203, -46.0012) -> (5.4973, -46.5388)
  arc A93 (5.7078, -46.8395) -> (5.4973, -46.5388) centre (5.3878, -46.8395) ccw
  line L190 (5.7078, -46.8395) -> (5.7078, -46.887)
  arc A94 (5.4973, -47.1877) -> (5.7078, -46.887) centre (5.3878, -46.887) ccw
  line L191 (5.4973, -47.1877) -> (4.0203, -47.7253)
  line L192 (4.0203, -47.7253) -> (4.0203, -48.3574)
  line L193 (4.0203, -48.3574) -> (5.4973, -48.895)
  arc A95 (5.7078, -49.1957) -> (5.4973, -48.895) centre (5.3878, -49.1957) ccw
  line L194 (5.7078, -49.1957) -> (5.7078, -49.2432)
  arc A96 (5.4973, -49.5439) -> (5.7078, -49.2432) centre (5.3878, -49.2432) ccw
  line L195 (5.4973, -49.5439) -> (4.0203, -50.0815)
  line L196 (4.0203, -50.0815) -> (4.0203, -50.7136)
  line L197 (4.0203, -50.7136) -> (5.4973, -51.2512)
  arc A97 (5.7078, -51.5519) -> (5.4973, -51.2512) centre (5.3878, -51.5519) ccw
  line L198 (5.7078, -51.5519) -> (5.7078, -51.5994)
  arc A98 (5.4973, -51.9001) -> (5.7078, -51.5994) centre (5.3878, -51.5994) ccw
  line L199 (5.4973, -51.9001) -> (4.0203, -52.4377)
  line L200 (4.0203, -52.4377) -> (4.0203, -53.0698)
  line L201 (4.0203, -53.0698) -> (5.4973, -53.6074)
  arc A99 (5.7078, -53.9081) -> (5.4973, -53.6074) centre (5.3878, -53.9081) ccw
  line L202 (5.7078, -53.9081) -> (5.7078, -53.9556)
  arc A100 (5.4973, -54.2563) -> (5.7078, -53.9556) centre (5.3878, -53.9556) ccw
  line L203 (5.4973, -54.2563) -> (4.0203, -54.7939)
  line L204 (4.0203, -54.7939) -> (4.0203, -55.426)
  line L205 (4.0203, -55.426) -> (5.4973, -55.9636)
  arc A101 (5.7078, -56.2643) -> (5.4973, -55.9636) centre (5.3878, -56.2643) ccw
  line L206 (5.7078, -56.2643) -> (5.7078, -56.3118)
  arc A102 (5.4973, -56.6125) -> (5.7078, -56.3118) centre (5.3878, -56.3118) ccw
  line L207 (5.4973, -56.6125) -> (4.0203, -57.1501)
  line L208 (4.0203, -57.1501) -> (4.0203, -57.7822)
  line L209 (4.0203, -57.7822) -> (5.4973, -58.3198)
  arc A103 (5.7078, -58.6205) -> (5.4973, -58.3198) centre (5.3878, -58.6205) ccw
  line L210 (5.7078, -58.6205) -> (5.7078, -58.668)
  arc A104 (5.4973, -58.9687) -> (5.7078, -58.668) centre (5.3878, -58.668) ccw
  line L211 (5.4973, -58.9687) -> (4.0203, -59.5063)
  line L212 (4.0203, -59.5063) -> (4.0203, -60.1384)
  line L213 (4.0203, -60.1384) -> (5.4973, -60.676)
  arc A105 (5.7078, -60.9767) -> (5.4973, -60.676) centre (5.3878, -60.9767) ccw
  line L214 (5.7078, -60.9767) -> (5.7078, -61.0242)
  arc A106 (5.4973, -61.3249) -> (5.7078, -61.0242) centre (5.3878, -61.0242) ccw
  line L215 (5.4973, -61.3249) -> (4.0203, -61.8625)
  line L216 (4.0203, -61.8625) -> (4.0203, -62.4946)
  line L217 (4.0203, -62.4946) -> (5.4973, -63.0322)
  arc A107 (5.7078, -63.3329) -> (5.4973, -63.0322) centre (5.3878, -63.3329) ccw
  line L218 (5.7078, -63.3329) -> (5.7078, -63.3804)
  arc A108 (5.4973, -63.6811) -> (5.7078, -63.3804) centre (5.3878, -63.3804) ccw
  line L219 (5.4973, -63.6811) -> (4.0203, -64.2187)
  line L220 (4.0203, -64.2187) -> (4.0203, -64.8508)
  line L221 (4.0203, -64.8508) -> (5.4973, -65.3884)
  arc A109 (5.7078, -65.6891) -> (5.4973, -65.3884) centre (5.3878, -65.6891) ccw
  line L222 (5.7078, -65.6891) -> (5.7078, -65.7366)
  arc A110 (5.4973, -66.0373) -> (5.7078, -65.7366) centre (5.3878, -65.7366) ccw
  line L223 (5.4973, -66.0373) -> (4.0203, -66.5748)
  line L224 (4.0203, -66.5748) -> (4.0203, -67.207)
  line L225 (4.0203, -67.207) -> (5.4973, -67.7446)
  arc A111 (5.7078, -68.0453) -> (5.4973, -67.7446) centre (5.3878, -68.0453) ccw
  line L226 (5.7078, -68.0453) -> (5.7078, -68.0928)
  arc A112 (5.4973, -68.3935) -> (5.7078, -68.0928) centre (5.3878, -68.0928) ccw
  line L227 (5.4973, -68.3935) -> (4.0203, -68.931)
  line L228 (4.0203, -68.931) -> (4.0203, -69.5632)
  line L229 (4.0203, -69.5632) -> (5.4973, -70.1007)
  arc A113 (5.7078, -70.4015) -> (5.4973, -70.1007) centre (5.3878, -70.4015) ccw
  line L230 (5.7078, -70.4015) -> (5.7078, -70.449)
  arc A114 (5.4973, -70.7497) -> (5.7078, -70.449) centre (5.3878, -70.449) ccw
  line L231 (5.4973, -70.7497) -> (4.0203, -71.2872)
  line L232 (4.0203, -71.2872) -> (4.0203, -71.9194)
  line L233 (4.0203, -71.9194) -> (5.4973, -72.4569)
  arc A115 (5.7078, -72.7576) -> (5.4973, -72.4569) centre (5.3878, -72.7576) ccw